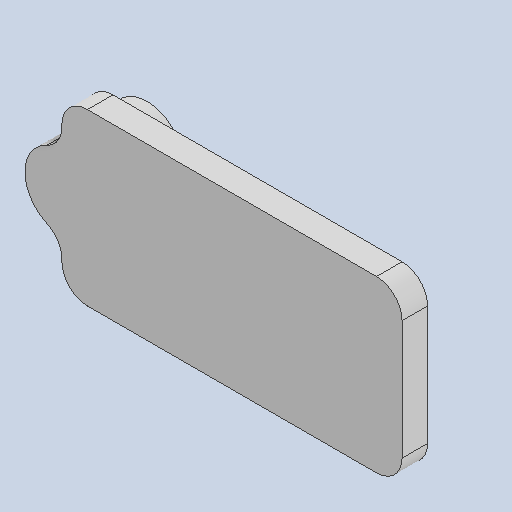
# Autodesk Inventor part: TutupTank
Saved by Autodesk Inventor 2026.2 (Build 302298010, 298A)
## iProperties
Created: 2026-05-22
Part Number: TutupTank
Material: Generic
Document SubType Name: Modeling
Designer: rizky
Density: 1 g/cm^3
Appearance: Default
Author: rizky
Autodesk Inventor part; units mm, degrees
ref_plane "YZ Plane" through (0, 0, 0) normal (1, 0, 0) x (0, 1, 0)
ref_plane "XZ Plane" through (0, 0, 0) normal (0, 1, 0) x (-1, 0, 0)
ref_plane "XY Plane" through (0, 0, 0) normal (0, 0, 1) x (1, 0, 0)
sketch "Sketch3" plane through (0, 0, 0) normal (0, 0, 1) x (1, 0, 0)
  circle A0 centre (0, 0) radius 2.35
  circle A1 centre (0, 0) radius 4.35
  dimension "d8" = 4.7
  dimension "d9" = 2
  constraints: 2 centre point, 1 coincident
  measures "d8" diameter of A0
  measures "d9" radial gap between concentric circles of A0 A1
extrude "Extrusion3" add sketch "Sketch3" against normal blind 10
sketch "Sketch4" plane through (0, 0, 0) normal (0, 0, 1) x (1, 0, 0)
  circle A0 centre (0, 0) radius 4.35 projected
  circle A1 centre (0, 0) radius 2.35 projected
  line L0 (0, 0) -> (40, 0)
  line L1 (40, 0) -> (40, 10)
  line L2 (40, 10) -> (0, 10)
  line L3 (0, 10) -> (0, 0)
  line L4 (40, 0) -> (40, -10)
  line L5 (40, -10) -> (0, -10)
  line L6 (0, -10) -> (0, 0)
  point P0 (0, 4.35)
  point P1 (0, -4.35)
  dimension "d12" = 40
  dimension "d13" = 10
  constraints: 14 end point, 2 parallel, 2 symmetric about line, 1 horizontal, 1 perpendicular
  measures "d12" distance of L2.end L1.end
  measures "d13" distance of L1.end L0.end
extrude "Extrusion4" add sketch "Sketch4" against normal blind 3 contours L0 L4 L5 L6 A0 | A0 L3 L2 L1 L0
fillet "Fillet1" radius 3 6 edges at (0, -4.35, -1.5) (0, 4.35, -1.5) (0, -10, -1.5) (0, 10, -1.5) (40, 10, -1.5) (40, -10, -1.5)
sketch "Sketch5" plane through (0, 0, 0) normal (0, 0, 1) x (1, 0, 0)
  circle A0 centre (0, 0) radius 2.35 projected
extrude "Extrusion5" add sketch "Sketch5" against normal blind 6.5
sketch "Sketch6" plane through (0, 0, -3) normal (0, 0, -1) x (-1, 0, 0)
  arc A0 (-40, -7) -> (-37, -10) centre (-37, -7) ccw projected
  line L0 (-37, -10) -> (-3, -10) projected
  arc A1 (-3, -10) -> (0, -7) centre (-3, -7) ccw projected
  line L1 (0, -7) -> (0, -6.7099) projected
  arc A2 (1.7755, -3.9712) -> (0, -6.7099) centre (3, -6.7099) ccw projected
  arc A3 (1.7755, 3.9712) -> (1.7755, -3.9712) centre (0, 0) ccw projected
  arc A4 (0, 6.7099) -> (1.7755, 3.9712) centre (3, 6.7099) ccw projected
  line L2 (0, 6.7099) -> (0, 7) projected
  arc A5 (0, 7) -> (-3, 10) centre (-3, 7) ccw projected
  line L3 (-3, 10) -> (-37, 10) projected
  arc A6 (-37, 10) -> (-40, 7) centre (-37, 7) ccw projected
  line L4 (-40, 7) -> (-40, -7) projected
  line L5 (-20, -10) -> (-20, 10)
  line L6 (-40, 0) -> (-20, 0)
  circle A7 centre (-30, 0) radius 5.279
  dimension "d19" = 10.558
  constraints: 5 midpoint, 4 end point, 1 centre point
  measures "d19" diameter of A7
body "Solid2"
